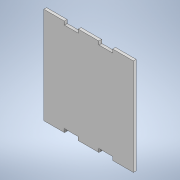
# Autodesk Inventor part: torso_base
Saved by Autodesk Inventor 2020.3 (Build 243373000, 373)
## iProperties
Created: 2020-08-06
Part Number: torso_base
Material: Generic
Document SubType Name: Modeling
Designer: aditk
Density: 1 g/cm^3
Appearance: Default
Author: aditk
Autodesk Inventor part; units mm, degrees
ref_plane "YZ Plane" through (0, 0, 0) normal (1, 0, 0) x (0, 1, 0)
ref_plane "XZ Plane" through (0, 0, 0) normal (0, 1, 0) x (-1, 0, 0)
ref_plane "XY Plane" through (0, 0, 0) normal (0, 0, 1) x (1, 0, 0)
sketch "Sketch1" plane through (0, 0, 0) normal (0, 0, 1) x (1, 0, 0)
  line L0 (65, -70) -> (65, 70)
  line L1 (-65, 70) -> (-65, -70)
  line L2 (-65, 70) -> (-65, 65)
  line L3 (-15, 65) -> (-15, 70)
  line L4 (-15, 65) -> (-35, 65)
  line L5 (-35, 65) -> (-35, 70)
  line L6 (15, 65) -> (15, 70)
  line L7 (35, 65) -> (35, 70)
  line L8 (-35, 70) -> (-65, 70)
  line L9 (65, 70) -> (35, 70)
  line L10 (15, 70) -> (-15, 70)
  line L11 (-15, -65) -> (-15, -70)
  line L12 (-15, -65) -> (-35, -65)
  line L13 (-35, -65) -> (-35, -70)
  line L14 (35, -65) -> (35, -70)
  line L15 (15, -65) -> (15, -70)
  line L16 (-35, -70) -> (-65, -70)
  line L17 (65, -70) -> (35, -70)
  line L18 (15, -70) -> (-15, -70)
  line L19 (-65, -70) -> (-35, -70)
  line L20 (35, -70) -> (65, -70)
  line L21 (-35, -65) -> (-15, -65)
  line L22 (15, -65) -> (35, -65)
  line L23 (-35, 65) -> (-15, 65)
  line L24 (15, 65) -> (35, 65)
  point P0 (0, 0)
  constraints: 50 end point, 9 perpendicular, 7 parallel, 2 horizontal, 1 point on line
extrude "Extrusion1" add sketch "Sketch1" along normal blind 4
sketch "Sketch2" plane through (-15, 70, 0) normal (0, 1, 0) x (1, 0, 0)
  line L0 (-20, 0) -> (-50, 0) projected
  line L1 (-50, 0) -> (-50, -4) projected
  line L2 (-20, -4) -> (-50, -4) projected
  line L3 (-20, 0) -> (-20, -4) projected
  line L4 (0, 0) -> (-20, 0) projected
  line L5 (-20, 0) -> (-20, -4) projected
  line L6 (0, -4) -> (-20, -4) projected
  line L7 (0, 0) -> (0, -4) projected
  line L8 (30, 0) -> (0, 0) projected
  line L9 (0, 0) -> (0, -4) projected
  line L10 (30, -4) -> (0, -4) projected
  line L11 (30, 0) -> (30, -4) projected
  line L12 (50, 0) -> (30, 0) projected
  line L13 (50, -4) -> (30, -4) projected
  line L14 (50, 0) -> (30, 0) projected
  line L15 (30, 0) -> (30, -4) projected
  line L16 (50, -4) -> (30, -4) projected
  line L17 (50, 0) -> (50, -4) projected
  line L18 (80, 0) -> (50, 0) projected
  line L19 (50, 0) -> (50, -4) projected
  line L20 (80, -4) -> (50, -4) projected
  line L21 (80, 0) -> (80, -4) projected
  point P0 (15, 0)
body "Solid1"
